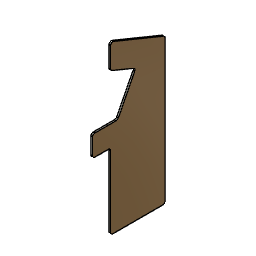
right_side_panel (Autodesk Fusion 360 design; units mm, degrees)
Autodesk Fusion 360 part; units mm, degrees
sketch "Side Panel" plane through (0, 0, 0) normal (1, 0, 0) x (0, 1, 0)
  line L0 (0, 0) -> (195, 0)
  line L1 (195, 0) -> (195, 520)
  line L2 (195, 520) -> (-0.3488, 600)
  line L3 (-0.3488, 600) -> (-0.3488, 510)
  line L4 (-0.3488, 510) -> (90, 473)
  line L5 (90, 473) -> (25, 345)
  line L6 (25, 345) -> (-65, 345)
  line L7 (-65, 345) -> (-65, 270)
  line L8 (-65, 270) -> (0, 270)
  line L9 (0, 270) -> (0, 0)
  dimension "d7" = 600
  dimension "d10" = 195
  dimension "d12" = 520
  dimension "d14" = 90
  dimension "d16" = 105
  dimension "d18" = 270
  dimension "d20" = 75
  dimension "d22" = 37
  dimension "d27" = 260
  dimension "d28" = 90
  dimension "d31" = 345
  constraint coincident L0.start L9.end
  constraint horizontal L0
  constraint perpendicular L0 L1
  constraint parallel L1 L3
  constraint parallel L2 L4
  constraint parallel L3 L7
  constraint perpendicular L7 L8
  constraint perpendicular L0 L9
  measures "d7" distance of L0 L2.end
  measures "d10" distance of L0.start L0.end
  measures "d12" distance of L0.end L1.end
  measures "d14" distance of L2.end L3.end
  measures "d16" distance of L1 L4.end
  measures "d18" distance of L8.end L0.start
  measures "d20" distance of L6.end L7.end
  measures "d22" vertical distance of L3.end L4.end
  measures "d27" distance of L1 L7
  measures "d28" horizontal distance of L5.end L6.end
  measures "d31" vertical distance of L0.start L5.end
extrude "Extrude1" add sketch "Side Panel" along normal blind 6 makes body 1
fillet "Fillet1" radius 8 10 edges at (3, -65, 345) (3, 25, 345) (3, 90, 473) (3, -0.3488, 510) (3, -0.3488, 600) (3, 195, 520) (3, -65, 270) (3, 0, 270) (3, 0, 0) (3, 195, 0) on bodies 1
sketch "Paint border" plane through (6, 0, 0) normal (1, 0, 0) x (0, 1, 0)
  arc A0 (187, 0) -> (195, 8) centre (187, 8) ccw
  line L0 (195, 8) -> (195, 514.6313)
  arc A1 (195, 514.6313) -> (190.0318, 522.0346) centre (187, 514.6313) ccw
  line L1 (190.0318, 522.0346) -> (10.683, 595.4822)
  arc A2 (10.683, 595.4822) -> (-0.3488, 588.079) centre (7.6512, 588.079) ccw
  line L2 (-0.3488, 588.079) -> (-0.3488, 515.3687)
  arc A3 (-0.3488, 515.3687) -> (4.6194, 507.9654) centre (7.6512, 515.3687) ccw
  line L3 (4.6194, 507.9654) -> (81.9699, 476.2885)
  arc A4 (86.0711, 465.263) -> (81.9699, 476.2885) centre (78.9381, 468.8853) ccw
  line L4 (86.0711, 465.263) -> (27.2231, 349.3778)
  arc A5 (20.0901, 345) -> (27.2231, 349.3778) centre (20.0901, 353) ccw
  line L5 (20.0901, 345) -> (-57, 345)
  arc A6 (-57, 345) -> (-65, 337) centre (-57, 337) ccw
  line L6 (-65, 337) -> (-65, 278)
  arc A7 (-65, 278) -> (-57, 270) centre (-57, 278) ccw
  line L7 (-57, 270) -> (-8, 270)
  arc A8 (0, 262) -> (-8, 270) centre (-8, 262) ccw
  line L8 (0, 262) -> (0, 8)
  arc A9 (0, 8) -> (8, 0) centre (8, 8) ccw
  line L9 (8, 0) -> (187, 0)
  line L10 (10, 6) -> (185, 6)
  line L11 (10, 6) -> (10, 280)
  line L12 (10, 280) -> (-55, 280)
  line L13 (-55, 280) -> (-55, 335)
  line L14 (-55, 335) -> (31.1374, 335)
  line L15 (9.6512, 516.7108) -> (103.8274, 478.1434)
  line L16 (31.1374, 335) -> (103.8274, 478.1434)
  line L17 (187.0159, 512.4636) -> (185, 6)
  line L18 (9.6512, 585.0987) -> (187.0159, 512.4636)
  line L19 (9.6512, 585.0987) -> (9.6512, 516.7108)
  dimension "d32" = 6
  dimension "d33" = 10
  dimension "d34" = 10
  dimension "d35" = 10
  dimension "d36" = 10
  dimension "d37" = 10
  dimension "d41" = 10
  dimension "d42" = 10
  dimension "d43" = 10
  dimension "d44" = 10
  constraint perpendicular L8 L10
  constraint perpendicular L10 L11
  constraint perpendicular L11 L12
  constraint perpendicular L12 L13
  constraint perpendicular L13 L14
  constraint parallel L3 L15
  constraint parallel L4 L16
  measures "d32" distance of L9 L10
  measures "d33" distance of L0 L10.end
  measures "d34" distance of L8 L10.start
  measures "d35" distance of L7 L11.end
  measures "d36" distance of L6 L12.end
  measures "d37" distance of L5 L13.end
  measures "d41" distance of L3 L15
  measures "d42" distance of L4 L16
  measures "d43" distance of L1 L18
  measures "d44" distance of L2 L19
extrude "Extrude2" cut sketch "Paint border" against normal blind 0.1 bodies 1
mirror "Mirror1" about plane through (0, 0, 0) normal (1, 0, 0) of bodies 1 makes body 2
hidden bodies 1
equation "MDFThickness = 6 mm" comment "Thickness of the MDF board"
equation "filletRadius = 8 mm" comment "Radius of all of the fillets on the side panel"
equation "d3 = MDFThickness"
equation "d6 = filletRadius"
equation "d7 = totaHeight"
equation "totaHeight = 600 mm" comment "Total height of the Smartie Sorrter"
equation "baseWidth = 195 mm" comment "Length of the bottom side of the side panel"
equation "d10 = baseWidth"
equation "backHight = 520 mm" comment "Height of the back side of the side panel"
equation "d12 = backHight"
equation "namePanelHeight = 90 mm" comment "Height of the top section containing the name panel"
equation "d14 = namePanelHeight"
equation "neckWidth = 105 mm" comment "Width of the neck between the bottom and top section"
equation "d16 = neckWidth"
equation "bottomFrontHeight = 270 mm" comment "Height of the bottom front section"
equation "d18 = bottomFrontHeight"
equation "controlPanelHeight = 75 mm" comment "Height of the control panel on the front"
equation "d20 = controlPanelHeight"
equation "namePanelFrontDipHeight = 37 mm" comment "Dip height on the front side below the name panel"
equation "d22 = namePanelFrontDipHeight"
equation "controlPanelTopWidth = 90 mm" comment "Top width of the control panel from the front to the viewing area"
equation "controlPanelTotalWidth = 260 mm" comment "Total width of the control panel area from the front to the back"
equation "d27 = controlPanelTotalWidth"
equation "d28 = controlPanelTopWidth"
equation "d31 = bottomFrontHeight + controlPanelHeight"
named bodies: "Left Side Panel", "Right Side Panel"
